Autodesk Inventor part; units mm, degrees
(part 4 of 4)
  arc A259 (62.7055, 12.3) -> (64.9055, 14.5) centre (62.7055, 14.5) ccw
  arc A260 (59.4055, -12.3) -> (57.2055, -14.5) centre (59.4055, -14.5) ccw
  line L401 (59.4055, -12.3) -> (62.7055, -12.3)
  arc A261 (64.9055, -14.5) -> (62.7055, -12.3) centre (62.7055, -14.5) ccw
  line L402 (57.2055, -25.5) -> (57.2055, -14.5)
  line L403 (62.7055, -27.7) -> (59.4055, -27.7)
  arc A262 (57.2055, -25.5) -> (59.4055, -27.7) centre (59.4055, -25.5) ccw
  line L404 (64.9055, -14.5) -> (64.9055, -25.5)
  line L405 (64.9055, -27.7) -> (57.2055, -12.3) construction
  line L406 (57.2055, -27.7) -> (64.9055, -12.3) construction
  arc A263 (62.7055, -27.7) -> (64.9055, -25.5) centre (62.7055, -25.5) ccw
  arc A264 (59.4055, 7.7) -> (57.2055, 5.5) centre (59.4055, 5.5) ccw
  line L407 (59.4055, 7.7) -> (62.7055, 7.7)
  arc A265 (64.9055, 5.5) -> (62.7055, 7.7) centre (62.7055, 5.5) ccw
  line L408 (57.2055, -5.5) -> (57.2055, 5.5)
  line L409 (62.7055, -7.7) -> (59.4055, -7.7)
  arc A266 (57.2055, -5.5) -> (59.4055, -7.7) centre (59.4055, -5.5) ccw
  line L410 (64.9055, 5.5) -> (64.9055, -5.5)
  line L411 (64.9055, -7.7) -> (57.2055, 7.7) construction
  line L412 (57.2055, -7.7) -> (64.9055, 7.7) construction
  arc A267 (62.7055, -7.7) -> (64.9055, -5.5) centre (62.7055, -5.5) ccw
  line L413 (63.7413, -39.95) -> (58.1413, -39.95)
  line L414 (55.9413, -37.75) -> (55.9413, -37.15)
  line L415 (58.1413, -34.95) -> (63.7413, -34.95)
  line L416 (65.9413, -37.15) -> (65.9413, -37.75)
  line L417 (65.9413, -39.95) -> (55.9413, -34.95) construction
  line L418 (55.9413, -39.95) -> (65.9413, -34.95) construction
  arc A268 (65.9413, -37.15) -> (63.7413, -34.95) centre (63.7413, -37.15) ccw
  arc A269 (63.7413, -39.95) -> (65.9413, -37.75) centre (63.7413, -37.75) ccw
  arc A270 (55.9413, -37.75) -> (58.1413, -39.95) centre (58.1413, -37.75) ccw
  arc A271 (58.1413, -34.95) -> (55.9413, -37.15) centre (58.1413, -37.15) ccw
  line L419 (55.9413, 37.75) -> (55.9413, 37.15)
  arc A272 (55.9413, 37.15) -> (58.1413, 34.95) centre (58.1413, 37.15) ccw
  arc A273 (58.1413, 39.95) -> (55.9413, 37.75) centre (58.1413, 37.75) ccw
  line L420 (63.7413, 39.95) -> (58.1413, 39.95)
  line L421 (58.1413, 34.95) -> (63.7413, 34.95)
  line L422 (65.9413, 39.95) -> (55.9413, 34.95) construction
  line L423 (55.9413, 39.95) -> (65.9413, 34.95) construction
  arc A274 (63.7413, 34.95) -> (65.9413, 37.15) centre (63.7413, 37.15) ccw
  line L424 (65.9413, 37.15) -> (65.9413, 37.75)
  arc A275 (65.9413, 37.75) -> (63.7413, 39.95) centre (63.7413, 37.75) ccw
  point P0 (-42.4088, 42.409)
  point P1 (-28.2667, 28.2668)
  point P2 (-14.1246, 14.1246)
  point P3 (-0.0083, 64.091)
  point P4 (19.9917, 64.091)
  point P5 (39.9917, 64.091)
  point P6 (-20.0083, 64.091)
  point P7 (-0.0083, 64.091)
  point P8 (19.9917, 64.091)
  point P9 (-40.0083, 64.091)
  point P10 (-20.0083, 64.091)
  point P11 (-0.0083, 64.091)
  point P12 (-0.0083, -64.091)
  point P13 (19.9917, -64.091)
  point P14 (39.9917, -64.091)
  point P15 (-20.0083, -64.091)
  point P16 (-0.0083, -64.091)
  point P17 (19.9917, -64.091)
  point P18 (-40.0083, -64.091)
  point P19 (-20.0083, -64.091)
  point P20 (-0.0083, -64.091)
  point P21 (-14.1246, -14.1246)
  point P22 (19.3996, -4.4032)
  point P23 (50.0055, 35.0476)
  point P24 (19.3996, 4.4418)
  point P25 (4.0012, -18.9084)
  point P26 (42.4088, 42.409)
  point P27 (28.2667, 28.2668)
  point P28 (14.1246, 14.1246)
  point P29 (40.7278, 40.728)
  point P30 (14.1246, -14.1246)
  point P31 (40.7278, -40.728)
  point P32 (34.2063, -39.6512)
  point P33 (50.6112, -45.1667)
  point P34 (-61.9413, -61.941)
  point P35 (61.9413, -61.941)
  point P36 (0, 12.41)
  point P37 (0, 24.82)
  point P38 (0, 37.23)
  point P39 (0, 49.64)
  point P40 (0, -12.41)
  point P41 (0, 12.41)
  point P42 (0, 24.82)
  point P43 (0, 37.23)
  point P44 (0, -24.82)
  point P45 (0, -12.41)
  point P46 (0, 12.41)
  point P47 (0, 24.82)
  point P48 (0, -37.23)
  point P49 (0, -24.82)
  point P50 (0, -12.41)
  point P51 (0, 12.41)
  point P52 (0, -49.64)
  point P53 (0, -37.23)
  point P54 (0, -24.82)
  point P55 (0, -12.41)
  point P56 (-61.0555, 0)
  point P57 (-61.0555, 20)
  point P58 (-61.0555, -20)
  point P59 (-61.0555, 0)
  point P60 (-60.9413, -37.45)
  point P61 (-60.9413, 37.45)
  point P62 (61.0555, 0)
  point P63 (61.0555, 20)
  point P64 (61.0555, -20)
  point P65 (61.0555, 0)
  point P66 (60.9413, -37.45)
  point P67 (60.9413, 37.45)
  dimension "d6" = 4.2
  dimension "d7" = 10.9
  dimension "d8" = 10.9
  dimension "d9" = 15.5
  dimension "d10" = 7.7
  dimension "d11" = 18.6
  dimension "d12" = 2
  dimension "d15" = 20
  dimension "d20" = 64.233
  dimension "d21" = 15.4
  dimension "d22" = 7.7
  dimension "d23" = 4
  dimension "d24" = 2
  dimension "d27" = 20
  dimension "d30" = 20
  dimension "d35" = 5
  dimension "d36" = 8.9
  dimension "d37" = 1.2
  dimension "d40" = 12.41
  dimension "d43" = 12.41
  dimension "d46" = 7.7
  dimension "d47" = 15.4
  dimension "d48" = 7.2
  dimension "d49" = 2.2
  dimension "d52" = 20
  dimension "d55" = 20
  dimension "d58" = 10
  dimension "d59" = 5
  dimension "d60" = 7.25
  dimension "d61" = 6
  dimension "d62" = 2.2
  constraints: 836 end point, 543 point on line, 537 point on circle, 448 symmetric about line, 274 centre point, 130 midpoint, 40 tangent, 15 equal radius, 11 parallel, 8 perpendicular, 5 horizontal, 4 vertical, 1 collinear, 1109 other
  measures "d6" diameter of A1
  measures "d7" distance from line of L3 A1.centre
  measures "d8" distance from line of L2 A1.centre
  measures "d9" distance between parallel lines of L9 L7
  measures "d10" distance between parallel lines of L8 L6
  measures "d11" distance from line of A1.centre L7
  measures "d12" radius of A2
  measures "d15" distance of A2.centre A6.centre
  measures "d20" distance between parallel lines of L3 L29
  measures "d21" distance between parallel lines of L27 L29
  measures "d22" distance between parallel lines of L28 L26
  measures "d23" distance between parallel lines of L2 L28
  measures "d24" radius of A14
  measures "d27" distance of L28.start L36.start
  measures "d30" distance of L28.start L48.start
  measures "d35" diameter of A126
  measures "d36" distance from line of L198 A126.centre
  measures "d37" radius of A128
  measures "d40" distance of L203.start L209.start
  measures "d43" distance of L203.start L233.start
  measures "d46" distance of L355.end L356.end
  measures "d47" distance of L356.end L355.start
  measures "d48" distance between parallel lines of L350 L352
  measures "d49" radius of A228
  measures "d52" distance of A229.centre A233.centre
  measures "d55" distance of A229.centre A237.centre
  measures "d58" distance between parallel lines of L376 L378
  measures "d59" distance between parallel lines of L375 L377
  measures "d60" distance between parallel lines of L363 L377
  measures "d61" distance between parallel lines of L3 L378
  measures "d62" radius of A244
extrude "Extrusion2" cut sketch "Sketch4" against normal through all
body "Solid1"
